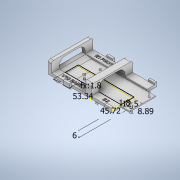
# Autodesk Inventor part: R1 Proto V10 Base
Saved by Autodesk Inventor 2021 (Build 250183000, 183)
## iProperties
Created: 2020-06-07
Part Number: R1 Proto V10 Base
Material: Generic
Document SubType Name: Modeling
Designer: andre
Density: 1 g/cm^3
Appearance: Default
Author: andre
## iProperties of the stored document _3DPrint.ipt
Created: 2020-06-07
Part Number: _3DPrint
Material: Generic
Document SubType Name: Modeling
Designer: andre
Density: 1 g/cm^3
Appearance: Default
Author: andre
Autodesk Inventor part; units mm, degrees
ref_plane "YZ Plane" through (0, 0, 0) normal (1, 0, 0) x (0, 1, 0)
ref_plane "XZ Plane" through (0, 0, 0) normal (0, 1, 0) x (-1, 0, 0)
ref_plane "XY Plane" through (0, 0, 0) normal (0, 0, 1) x (1, 0, 0)
sketch "Sketch1" plane through (0, 0, 0) normal (0, 1, 0) x (-1, 0, 0)
  line L0 (0, 0) -> (62, 0)
  line L1 (62, 0) -> (62, -19.7)
  line L2 (62, -19.7) -> (0, -19.7)
  line L3 (0, -19.7) -> (0, 0)
  dimension "d5" = 62
  dimension "d6" = 19.7
  constraints: 8 end point, 2 parallel, 1 horizontal, 1 perpendicular
  measures "d5" distance of L1.end L2.end
  measures "d6" distance of L0.end L1.end
extrude "Extrusion1" add sketch "Sketch1" along normal blind 2.4
sketch "Sketch3" plane through (-62, 0, 0) normal (0, 0, 1) x (1, 0, 0)
  line L0 (62, 2.4) -> (0, 2.4) projected
  line L1 (62, 0) -> (0, 0) projected
  line L2 (62, 2.4) -> (56, 2.4)
  line L3 (56, 2.4) -> (56, 0)
  line L4 (56, 0) -> (62, 0)
  line L5 (62, 0) -> (62, 2.4)
  line L6 (22, 2.4) -> (22, 0) construction
  line L7 (22, 2.4) -> (16, 2.4)
  line L8 (16, 2.4) -> (16, 0)
  line L9 (16, 0) -> (22, 0)
  line L10 (22, 0) -> (22, 2.4)
  point P0 (62, 0)
  point P1 (22, 0)
  dimension "d9" = 6
  dimension "d13" = 6
  dimension "d14" = 34
  dimension "d79" = 2.4
  constraints: 18 end point, 4 parallel, 4 point on line, 3 perpendicular, 2 horizontal
  measures "d9" distance of L4.end L3.end
  measures "d13" distance of L9.end L8.end
  measures "d14" distance between parallel lines of L3 L6
  measures "d79" distance between parallel lines of L1 L0
extrude "Extrusion2" add sketch "Sketch3" along normal blind 2 contours L5 L1 L3 L0 | L10 L1 L8 L0
ref_plane "Work Plane1" through (0, 0, -19.7) normal (0, 0, -1) x (-1, 0, 0)
sketch "Sketch4" plane through (0, 2.4, 0) normal (0, 1, 0) x (1, 0, 0)
  line L0 (-6, -2) -> (0, -2) projected
  line L1 (-6, -2) -> (0, -2)
  line L2 (0, -2) -> (0, 0)
  line L3 (0, 0) -> (-6, 0)
  line L4 (-6, 0) -> (-6, -2)
  line L5 (-46, -2) -> (-40, -2) projected
  line L6 (-40, 0) -> (-40, -2) projected
  line L7 (-46, -2) -> (-40, -2)
  line L8 (-40, -2) -> (-40, 0)
  line L9 (-40, 0) -> (-46, 0)
  line L10 (-46, 0) -> (-46, -2)
  constraints: 16 end point, 4 parallel, 2 horizontal, 2 perpendicular
extrude "Extrusion3" add sketch "Sketch4" along normal blind 1.6
sketch "Sketch5" plane through (0, 2.4, 0) normal (0, 1, 0) x (1, 0, 0)
  point P0 (0, 0)
sketch "Sketch6" plane through (0, 2.4, 0) normal (0, 1, 0) x (1, 0, 0)
  line L0 (0, 19.7) -> (-62, 19.7) projected
  line L1 (-40, 0) -> (-6, 0) projected
  line L2 (-21, 19.7) -> (-27, 19.7)
  line L3 (-27, 19.7) -> (-27, 0)
  line L4 (-27, 0) -> (-21, 0)
  line L5 (-21, 0) -> (-21, 19.7)
  line L6 (0, 19.7) -> (0, 0) projected
  dimension "d18" = 6
  dimension "d19" = 21
  constraints: 8 end point, 2 parallel, 2 point on line, 1 horizontal, 1 perpendicular
  measures "d18" distance of L4.end L3.end
  measures "d19" distance between parallel lines of L6 L5
extrude "Extrusion4" add sketch "Sketch6" along normal blind 9.6
sketch "Sketch7" plane through (-21, 2.4, 0) normal (1, 0, 0) x (0, 0, -1)
  point P0 (0, -2.4)
sketch "Sketch8" plane through (-21, 2.4, 0) normal (1, 0, 0) x (0, 0, -1)
  line L0 (19.7, 0) -> (19.7, 9.6) projected
  line L1 (19.7, 0) -> (7.2, 0)
  line L2 (7.2, 0) -> (7.2, 8.1)
  line L3 (7.2, 8.1) -> (19.7, 8.1)
  line L4 (19.7, 8.1) -> (19.7, 0)
  line L5 (0, 0) -> (0, 9.6) projected
  line L6 (19.7, 0) -> (0, 0) projected
  line L7 (0, 9.6) -> (19.7, 9.6) projected
  point P0 (0, -2.4)
  point P1 (19.7, 8.1)
  dimension "d22" = 19.7
  dimension "d23" = 9.6
  dimension "d24" = 12.5
  dimension "d25" = 8.1
  constraints: 8 end point, 2 parallel, 1 horizontal, 1 perpendicular
  measures "d22" distance between parallel lines of L0 L5
  measures "d23" distance between parallel lines of L6 L7
  measures "d24" distance between parallel lines of L0 L2
  measures "d25" distance between parallel lines of L1 L3
extrude "Extrusion5" cut sketch "Sketch8" against normal blind 37.6 contours L1 L2 L3 L0
ref_plane "Work Plane2" through (-43, 0, -19.7) normal (-1, 0, 0) x (0, 0, 1)
mirror "Mirror2" about plane through (-43, 0, -19.7) normal (-1, 0, 0) of "Extrusion4", "Extrusion5"
sketch "Sketch12" plane through (0, 2.4, 0) normal (0, 1, 0) x (1, 0, 0)
  line L0 (0, 19.7) -> (0, -2) projected
  line L1 (0, 19.7) -> (-53.34, 19.7)
  line L2 (-53.34, 19.7) -> (-53.34, 7.2)
  line L3 (-53.34, 7.2) -> (0, 7.2)
  line L4 (0, 7.2) -> (0, 19.7)
  point P0 (0, 0)
  point P1 (0, 7.2)
  dimension "d41" = 53.34
  dimension "d42" = 12.5
  constraints: 8 end point, 2 parallel, 1 horizontal, 1 perpendicular
  measures "d41" distance between parallel lines of L2 L0
  measures "d42" distance between parallel lines of L1 L3
extrude "Extrusion8" cut sketch "Sketch12" against normal blind 1.4
fillet "Fillet3" radius 2 2 edges at (-62, 12, 0) (-24, 12, 0) curvature continuous yes
fillet "Fillet4" radius 7 2 edges at (-62, 10.5, -7.2) (-24, 10.5, -7.2) curvature continuous yes
sketch "Sketch13" plane through (0, 1, 0) normal (0, 1, 0) x (1, 0, 0)
  circle A0 centre (6, 10.81) radius 0.9
  circle A1 centre (-39.72, 12.1417) radius 0.9
  line L0 (-53.34, 19.7) -> (0, 19.7) projected
  line L1 (0, 19.7) -> (0, 7.2) projected
  point P0 (0, 0)
  dimension "d48" = 1.8
  dimension "d49" = 1.8
  dimension "d50" = 45.72
  dimension "d51" = 8.89
  dimension "d76" = 6
  constraints: 2 centre point
  measures "d48" diameter of A0
  measures "d49" diameter of A1
  measures "d50" horizontal distance of A1.centre A0.centre
  measures "d51" distance from line of L0 A0.centre
  measures "d76" distance from line of L1 A0.centre
extrude "Extrusion9" add sketch "Sketch13" along normal blind 4 contours A0
mirror "Mirror3" about plane through (0, 0, -19.7) normal (0, 0, -1) of "Extrusion4", "Extrusion5", "Mirror2", "Fillet4", "Fillet3", "Extrusion1", "Extrusion3", "Extrusion2", "Extrusion9", "Extrusion8"
sketch "Sketch14" plane through (-62, 0, 0) normal (-1, 0, 0) x (0, 0, 1)
  line L0 (-58.5888, -16.4354) -> (8.8289, -16.4354)
  line L1 (8.8289, -16.4354) -> (8.8289, 25.7982)
  line L2 (8.8289, 25.7982) -> (-58.5888, 25.7982)
  line L3 (-58.5888, 25.7982) -> (-58.5888, -16.4354)
  point P0 (0, 0)
  constraints: 8 end point, 2 parallel, 1 horizontal, 1 perpendicular
extrude "Extrusion10" cut sketch "Sketch14" along normal blind 5
chamfer "Chamfer1" distance 5 distance2 1.4 1 edges at (-53.34, 2.4, -19.7) measured on face at (-53.84, 2.4, -19.7)
sketch "Sketch15" plane through (0, 2.4, 0) normal (0, 1, 0) x (1, 0, 0)
  line L0 (-57, 38.4) -> (-29, 38.4) construction
  line L1 (-29, 38.4) -> (-29, 33.2) construction
  line L2 (-29, 33.2) -> (-57, 33.2) construction
  line L3 (-57, 33.2) -> (-57, 38.4) construction
  line L4 (-59, 37.4) -> (-59, 2) projected
  line L5 (-27, 2) -> (-27, 37.4) projected
  line L6 (-59, 39.4) -> (-46, 39.4) projected
  line L7 (-58.34, 32.2) -> (0, 32.2) projected
  line L8 (-57, 6.2) -> (-29, 6.2) construction
  line L9 (-29, 6.2) -> (-29, 1) construction
  line L10 (-29, 1) -> (-57, 1) construction
  line L11 (-57, 1) -> (-57, 6.2) construction
  line L12 (0, 7.2) -> (-58.34, 7.2) projected
  line L13 (-59, 0) -> (-46, 0) projected
  line L14 (-14.9129, 6.2) -> (-6.0871, 6.2) construction
  line L15 (-6.0871, 6.2) -> (-6.0871, 1) construction
  line L16 (-6.0871, 1) -> (-14.9129, 1) construction
  line L17 (-14.9129, 1) -> (-14.9129, 6.2) construction
  line L18 (-21, 2) -> (-21, 37.4) projected
  line L19 (0, 7.2) -> (0, 0) projected
  spline S0 degree 2 poles (-51.0157, 2.1) (-50.8394, 2.1) (-50.6147, 2.2691) (-50.5495, 2.4527) knots 0 0 0 1 2 2 2
  line L20 (-50.5495, 2.4527) -> (-49.7307, 4.6556)
  spline S1 degree 2 poles (-49.7307, 4.6556) (-49.7017, 4.7377) (-49.7017, 4.8174) knots 0 0 0 1 1 1
  spline S2 degree 2 poles (-49.7017, 4.8174) (-49.7041, 4.9454) (-49.8732, 5.0976) (-50.0157, 5.1) knots 0 0 0 1 2 2 2
  spline S3 degree 2 poles (-50.0157, 5.1) (-50.1341, 5.1) (-50.279, 4.9865) (-50.3176, 4.8657) knots 0 0 0 1 2 2 2
  line L21 (-50.3176, 4.8657) -> (-50.9988, 2.7691)
  line L22 (-50.9988, 2.7691) -> (-51.0133, 2.7691)
  line L23 (-51.0133, 2.7691) -> (-51.6969, 4.8585)
  spline S4 degree 2 poles (-51.6969, 4.8585) (-51.7331, 4.9841) (-51.8853, 5.1) (-52.0085, 5.1) knots 0 0 0 1 2 2 2
  spline S5 degree 2 poles (-52.0085, 5.1) (-52.1558, 5.0976) (-52.3273, 4.9406) (-52.3297, 4.8101) knots 0 0 0 1 2 2 2
  spline S6 degree 2 poles (-52.3297, 4.8101) (-52.3297, 4.7232) (-52.3007, 4.6386) knots 0 0 0 1 1 1
  line L24 (-52.3007, 4.6386) -> (-51.4867, 2.4551)
  spline S7 degree 2 poles (-51.4867, 2.4551) (-51.4215, 2.2691) (-51.1944, 2.1) (-51.0157, 2.1) knots 0 0 0 1 2 2 2
  spline S8 degree 2 poles (-48.3708, 2.0952) (-48.2331, 2.0976) (-48.0713, 2.2618) (-48.0688, 2.4019) knots 0 0 0 1 2 2 2
  line L25 (-48.0688, 2.4019) -> (-48.0688, 4.7618)
  spline S9 degree 2 poles (-48.0688, 4.7618) (-48.0713, 4.9213) (-48.2524, 5.1024) (-48.4167, 5.1048) knots 0 0 0 1 2 2 2
  spline S10 degree 2 poles (-48.4167, 5.1048) (-48.5085, 5.1048) (-48.6751, 5.0589) (-48.779, 4.9889) knots 0 0 0 1 2 2 2
  line L26 (-48.779, 4.9889) -> (-49.3587, 4.5879)
  spline S11 degree 2 poles (-49.3587, 4.5879) (-49.4287, 4.5372) (-49.4915, 4.4285) (-49.4915, 4.3585) knots 0 0 0 1 2 2 2
  spline S12 degree 2 poles (-49.4915, 4.3585) (-49.4891, 4.2594) (-49.3708, 4.1411) (-49.2766, 4.1411) knots 0 0 0 1 2 2 2
  spline S13 degree 2 poles (-49.2766, 4.1411) (-49.2307, 4.1411) (-49.1558, 4.1652) (-49.1147, 4.1942) knots 0 0 0 1 2 2 2
  line L27 (-49.1147, 4.1942) -> (-48.6872, 4.4937)
  line L28 (-48.6872, 4.4937) -> (-48.6751, 4.4937)
  line L29 (-48.6751, 4.4937) -> (-48.6751, 2.4019)
  spline S14 degree 2 poles (-48.6751, 2.4019) (-48.6727, 2.2618) (-48.5085, 2.0976) (-48.3708, 2.0952) knots 0 0 0 1 2 2 2
  spline S15 degree 2 poles (-46.2597, 2.0734) (-45.8877, 2.0758) (-45.3563, 2.4478) (-45.0713, 3.1314) (-45.0688, 3.6072) knots 0 0 0 1 2 3 3 3
  spline S16 degree 2 poles (-45.0688, 3.6072) (-45.0713, 4.0807) (-45.3563, 4.7594) (-45.8901, 5.1242) (-46.2597, 5.1266) knots 0 0 0 1 2 3 3 3
  spline S17 degree 2 poles (-46.2597, 5.1266) (-46.6292, 5.1242) (-47.163, 4.757) (-47.4505, 4.0783) (-47.4505, 3.6048) knots 0 0 0 1 2 3 3 3
  spline S18 degree 2 poles (-47.4505, 3.6048) (-47.4505, 3.129) (-47.163, 2.4454) (-46.6316, 2.0758) (-46.2597, 2.0734) knots 0 0 0 1 2 3 3 3
  spline S19 degree 2 poles (-46.2597, 2.5638) (-46.5326, 2.5662) (-46.8273, 3.1) (-46.8297, 3.6048) knots 0 0 0 1 2 2 2
  spline S20 degree 2 poles (-46.8297, 3.6048) (-46.8273, 4.1048) (-46.5278, 4.6338) (-46.2597, 4.6362) knots 0 0 0 1 2 2 2
  spline S21 degree 2 poles (-46.2597, 4.6362) (-45.9891, 4.6338) (-45.692, 4.1048) (-45.6896, 3.6048) knots 0 0 0 1 2 2 2
  spline S22 degree 2 poles (-45.6896, 3.6048) (-45.692, 3.1) (-45.9867, 2.5662) (-46.2597, 2.5638) knots 0 0 0 1 2 2 2
  line L30 (-43.535, 2.1386) -> (-42.5471, 2.1386)
  spline S23 degree 2 poles (-42.5471, 2.1386) (-42.0737, 2.1435) (-41.5423, 2.5855) (-41.5374, 2.9744) knots 0 0 0 1 2 2 2
  spline S24 degree 2 poles (-41.5374, 2.9744) (-41.5423, 3.2691) (-41.9215, 3.6531) (-42.2258, 3.6821) knots 0 0 0 1 2 2 2
  line L31 (-42.2258, 3.6821) -> (-42.2258, 3.6966)
  spline S25 degree 2 poles (-42.2258, 3.6966) (-41.9867, 3.7377) (-41.6824, 4.0855) (-41.6775, 4.3319) knots 0 0 0 1 2 2 2
  spline S26 degree 2 poles (-41.6775, 4.3319) (-41.68, 4.67) (-42.1534, 5.0565) (-42.5688, 5.0589) knots 0 0 0 1 2 2 2
  line L32 (-42.5688, 5.0589) -> (-43.535, 5.0589)
  spline S27 degree 2 poles (-43.535, 5.0589) (-43.68, 5.0589) (-43.8394, 4.8923) (-43.8394, 4.7425) knots 0 0 0 1 2 2 2
  line L33 (-43.8394, 4.7425) -> (-43.8394, 2.4575)
  spline S28 degree 2 poles (-43.8394, 2.4575) (-43.8394, 2.3053) (-43.68, 2.1386) (-43.535, 2.1386) knots 0 0 0 1 2 2 2
  line L34 (-43.2283, 2.5952) -> (-43.2283, 3.443)
  line L35 (-43.2283, 3.443) -> (-42.7162, 3.443)
  spline S29 degree 2 poles (-42.7162, 3.443) (-42.4457, 3.4406) (-42.1606, 3.228) (-42.1606, 3.0227) knots 0 0 0 1 2 2 2
  spline S30 degree 2 poles (-42.1606, 3.0227) (-42.1606, 2.8126) (-42.4384, 2.5952) (-42.7041, 2.5952) knots 0 0 0 1 2 2 2
  line L36 (-42.7041, 2.5952) -> (-43.2283, 2.5952)
  line L37 (-43.2283, 3.844) -> (-43.2283, 4.6048)
  line L38 (-43.2283, 4.6048) -> (-42.7283, 4.6048)
  spline S31 degree 2 poles (-42.7283, 4.6048) (-42.5109, 4.6024) (-42.279, 4.4116) (-42.279, 4.2353) knots 0 0 0 1 2 2 2
  spline S32 degree 2 poles (-42.279, 4.2353) (-42.279, 4.0493) (-42.5447, 3.8464) (-42.7911, 3.844) knots 0 0 0 1 2 2 2
  line L39 (-42.7911, 3.844) -> (-43.2283, 3.844)
  spline S33 degree 2 poles (-40.994, 2.1) (-40.8732, 2.1) (-40.7258, 2.2304) (-40.6848, 2.3754) knots 0 0 0 1 2 2 2
  line L40 (-40.6848, 2.3754) -> (-40.5302, 2.8319)
  line L41 (-40.5302, 2.8319) -> (-39.4771, 2.8319)
  line L42 (-39.4771, 2.8319) -> (-39.3225, 2.3705)
  spline S34 degree 2 poles (-39.3225, 2.3705) (-39.2814, 2.228) (-39.1316, 2.1) (-39.0036, 2.1) knots 0 0 0 1 2 2 2
  spline S35 degree 2 poles (-39.0036, 2.1) (-38.8684, 2.1024) (-38.7017, 2.2594) (-38.6993, 2.3874) knots 0 0 0 1 2 2 2
  spline S36 degree 2 poles (-38.6993, 2.3874) (-38.6993, 2.4333) (-38.7162, 2.5227) (-38.7379, 2.5831) knots 0 0 0 1 2 2 2
  line L43 (-38.7379, 2.5831) -> (-39.5399, 4.7546)
  spline S37 degree 2 poles (-39.5399, 4.7546) (-39.6027, 4.9333) (-39.8273, 5.1) (-40.006, 5.1) knots 0 0 0 1 2 2 2
  spline S38 degree 2 poles (-40.006, 5.1) (-40.1775, 5.1) (-40.4022, 4.9309) (-40.465, 4.7546) knots 0 0 0 1 2 2 2
  line L44 (-40.465, 4.7546) -> (-41.2621, 2.5831)
  spline S39 degree 2 poles (-41.2621, 2.5831) (-41.2838, 2.5251) (-41.3031, 2.4261) (-41.3031, 2.3874) knots 0 0 0 1 2 2 2
  spline S40 degree 2 poles (-41.3031, 2.3874) (-41.3031, 2.2546) (-41.1389, 2.1024) (-40.994, 2.1) knots 0 0 0 1 2 2 2
  line L45 (-40.3973, 3.3053) -> (-40.0181, 4.501)
  line L46 (-40.0181, 4.501) -> (-40.0036, 4.501)
  line L47 (-40.0036, 4.501) -> (-39.6171, 3.3053)
  line L48 (-39.6171, 3.3053) -> (-40.3973, 3.3053)
  spline S41 degree 2 poles (-37.2597, 2.0903) (-36.7089, 2.0952) (-36.0882, 2.5879) (-36.0833, 3.0203) knots 0 0 0 1 2 2 2
  spline S42 degree 2 poles (-36.0833, 3.0203) (-36.0809, 3.3512) (-36.5085, 3.7473) (-36.9698, 3.8367) knots 0 0 0 1 2 2 2
  line L49 (-36.9698, 3.8367) -> (-37.279, 3.8995)
  spline S43 degree 2 poles (-37.279, 3.8995) (-37.535, 3.9502) (-37.7669, 4.1266) (-37.7645, 4.2594) knots 0 0 0 1 2 2 2
  spline S44 degree 2 poles (-37.7645, 4.2594) (-37.7597, 4.4237) (-37.4915, 4.6145) (-37.2621, 4.6169) knots 0 0 0 1 2 2 2
  spline S45 degree 2 poles (-37.2621, 4.6169) (-37.0737, 4.6169) (-36.7983, 4.4696) (-36.7258, 4.3053) knots 0 0 0 1 2 2 2
  spline S46 degree 2 poles (-36.7258, 4.3053) (-36.6751, 4.2111) (-36.535, 4.1242) (-36.4336, 4.1242) knots 0 0 0 1 2 2 2
  spline S47 degree 2 poles (-36.4336, 4.1242) (-36.3152, 4.1266) (-36.1751, 4.2594) (-36.1727, 4.3681) knots 0 0 0 1 2 2 2
  spline S48 degree 2 poles (-36.1727, 4.3681) (-36.1727, 4.4092) (-36.1848, 4.4744) (-36.1944, 4.5058) knots 0 0 0 1 2 2 2
  spline S49 degree 2 poles (-36.1944, 4.5058) (-36.2959, 4.7932) (-36.8563, 5.1072) (-37.2621, 5.1097) knots 0 0 0 1 2 2 2
  spline S50 degree 2 poles (-37.2621, 5.1097) (-37.5882, 5.1072) (-38.0906, 4.8874) (-38.3732, 4.4913) (-38.378, 4.2208) knots 0 0 0 1 2 3 3 3
  spline S51 degree 2 poles (-38.378, 4.2208) (-38.378, 3.8947) (-37.9457, 3.4792) (-37.5085, 3.3923) knots 0 0 0 1 2 2 2
  line L50 (-37.5085, 3.3923) -> (-37.1993, 3.3319)
  spline S52 degree 2 poles (-37.1993, 3.3319) (-36.9263, 3.2763) (-36.692, 3.0976) (-36.6944, 2.9551) knots 0 0 0 1 2 2 2
  spline S53 degree 2 poles (-36.6944, 2.9551) (-36.6993, 2.7908) (-36.9964, 2.5855) (-37.2452, 2.5831) knots 0 0 0 1 2 2 2
  spline S54 degree 2 poles (-37.2452, 2.5831) (-37.4577, 2.5807) (-37.7742, 2.7401) (-37.849, 2.9068) knots 0 0 0 1 2 2 2
  spline S55 degree 2 poles (-37.849, 2.9068) (-37.9022, 3.001) (-38.0374, 3.0855) (-38.1292, 3.0831) knots 0 0 0 1 2 2 2
  spline S56 degree 2 poles (-38.1292, 3.0831) (-38.25, 3.0831) (-38.3973, 2.9382) (-38.3998, 2.815) knots 0 0 0 1 2 2 2
  spline S57 degree 2 poles (-38.3998, 2.815) (-38.3998, 2.7739) (-38.3829, 2.6894) (-38.3659, 2.6507) knots 0 0 0 1 2 2 2
  spline S58 degree 2 poles (-38.3659, 2.6507) (-38.2766, 2.4068) (-37.7138, 2.0952) (-37.2597, 2.0903) knots 0 0 0 1 2 2 2
  line L51 (-35.407, 2.1386) -> (-34.0181, 2.1386)
  spline S59 degree 2 poles (-34.0181, 2.1386) (-33.8901, 2.1386) (-33.7428, 2.2715) (-33.7403, 2.3923) knots 0 0 0 1 2 2 2
  spline S60 degree 2 poles (-33.7403, 2.3923) (-33.7428, 2.5106) (-33.8925, 2.6435) (-34.0181, 2.6435) knots 0 0 0 1 2 2 2
  line L52 (-34.0181, 2.6435) -> (-35.1002, 2.6435)
  line L53 (-35.1002, 2.6435) -> (-35.1002, 3.3826)
  line L54 (-35.1002, 3.3826) -> (-34.0713, 3.3826)
  spline S61 degree 2 poles (-34.0713, 3.3826) (-33.9529, 3.3826) (-33.8176, 3.5058) (-33.8152, 3.6169) knots 0 0 0 1 2 2 2
  spline S62 degree 2 poles (-33.8152, 3.6169) (-33.8176, 3.7256) (-33.9553, 3.8512) (-34.0713, 3.8512) knots 0 0 0 1 2 2 2
  line L55 (-34.0713, 3.8512) -> (-35.1002, 3.8512)
  line L56 (-35.1002, 3.8512) -> (-35.1002, 4.5541)
  line L57 (-35.1002, 4.5541) -> (-34.0181, 4.5541)
  spline S63 degree 2 poles (-34.0181, 4.5541) (-33.8925, 4.5541) (-33.7428, 4.687) (-33.7403, 4.8053) knots 0 0 0 1 2 2 2
  spline S64 degree 2 poles (-33.7403, 4.8053) (-33.7428, 4.9261) (-33.8901, 5.0589) (-34.0181, 5.0589) knots 0 0 0 1 2 2 2
  line L58 (-34.0181, 5.0589) -> (-35.407, 5.0589)
  spline S65 degree 2 poles (-35.407, 5.0589) (-35.5519, 5.0589) (-35.7114, 4.8923) (-35.7114, 4.7425) knots 0 0 0 1 2 2 2
  line L59 (-35.7114, 4.7425) -> (-35.7114, 2.4575)
  spline S66 degree 2 poles (-35.7114, 2.4575) (-35.7114, 2.3053) (-35.5519, 2.1386) (-35.407, 2.1386) knots 0 0 0 1 2 2 2
  spline S67 degree 2 poles (-52.1534, 34.2952) (-52.0085, 34.2976) (-51.849, 34.4618) (-51.8466, 34.614) knots 0 0 0 1 2 2 2
  line L60 (-51.8466, 34.614) -> (-51.8466, 35.4063)
  line L61 (-51.8466, 35.4063) -> (-51.3273, 35.4063)
  line L62 (-51.3273, 35.4063) -> (-50.8418, 34.5271)
  spline S68 degree 2 poles (-50.8418, 34.5271) (-50.7717, 34.3966) (-50.6365, 34.2928) (-50.5302, 34.2952) knots 0 0 0 1 2 2 2
  spline S69 degree 2 poles (-50.5302, 34.2952) (-50.3949, 34.2976) (-50.2258, 34.4522) (-50.221, 34.5754) knots 0 0 0 1 2 2 2
  spline S70 degree 2 poles (-50.221, 34.5754) (-50.221, 34.6261) (-50.25, 34.7227) (-50.2862, 34.7855) knots 0 0 0 1 2 2 2
  line L63 (-50.2862, 34.7855) -> (-50.7089, 35.515)
  spline S71 degree 2 poles (-50.7089, 35.515) (-50.465, 35.6213) (-50.2065, 36.0512) (-50.2065, 36.329) knots 0 0 0 1 2 2 2
  spline S72 degree 2 poles (-50.2065, 36.329) (-50.2089, 36.7662) (-50.7548, 37.2541) (-51.2621, 37.2589) knots 0 0 0 1 2 2 2
  line L64 (-51.2621, 37.2589) -> (-52.1534, 37.2589)
  spline S73 degree 2 poles (-52.1534, 37.2589) (-52.2983, 37.2589) (-52.4577, 37.0923) (-52.4577, 36.9425) knots 0 0 0 1 2 2 2
  line L65 (-52.4577, 36.9425) -> (-52.4577, 34.614)
  spline S74 degree 2 poles (-52.4577, 34.614) (-52.4577, 34.4618) (-52.2983, 34.2976) (-52.1534, 34.2952) knots 0 0 0 1 2 2 2
  line L66 (-51.8466, 35.8507) -> (-51.8466, 36.7807)
  line L67 (-51.8466, 36.7807) -> (-51.3273, 36.7807)
  spline S75 degree 2 poles (-51.3273, 36.7807) (-51.0978, 36.7783) (-50.837, 36.5319) (-50.8345, 36.3169) knots 0 0 0 1 2 2 2
  spline S76 degree 2 poles (-50.8345, 36.3169) (-50.8345, 36.0971) (-51.0882, 35.8531) (-51.3225, 35.8507) knots 0 0 0 1 2 2 2
  line L68 (-51.3225, 35.8507) -> (-51.8466, 35.8507)
  spline S77 degree 2 poles (-48.8104, 34.2952) (-48.6727, 34.2976) (-48.5109, 34.4618) (-48.5085, 34.6019) knots 0 0 0 1 2 2 2
  line L69 (-48.5085, 34.6019) -> (-48.5085, 36.9618)
  spline S78 degree 2 poles (-48.5085, 36.9618) (-48.5109, 37.1213) (-48.692, 37.3024) (-48.8563, 37.3048) knots 0 0 0 1 2 2 2
  spline S79 degree 2 poles (-48.8563, 37.3048) (-48.9481, 37.3048) (-49.1147, 37.2589) (-49.2186, 37.1889) knots 0 0 0 1 2 2 2
  line L70 (-49.2186, 37.1889) -> (-49.7983, 36.7879)
  spline S80 degree 2 poles (-49.7983, 36.7879) (-49.8684, 36.7372) (-49.9312, 36.6285) (-49.9312, 36.5585) knots 0 0 0 1 2 2 2
  spline S81 degree 2 poles (-49.9312, 36.5585) (-49.9287, 36.4594) (-49.8104, 36.3411) (-49.7162, 36.3411) knots 0 0 0 1 2 2 2
  spline S82 degree 2 poles (-49.7162, 36.3411) (-49.6703, 36.3411) (-49.5954, 36.3652) (-49.5543, 36.3942) knots 0 0 0 1 2 2 2
  line L71 (-49.5543, 36.3942) -> (-49.1268, 36.6937)
  line L72 (-49.1268, 36.6937) -> (-49.1147, 36.6937)
  line L73 (-49.1147, 36.6937) -> (-49.1147, 34.6019)
  spline S83 degree 2 poles (-49.1147, 34.6019) (-49.1123, 34.4618) (-48.9481, 34.2976) (-48.8104, 34.2952) knots 0 0 0 1 2 2 2
  spline S84 degree 2 poles (-46.692, 34.3) (-46.5471, 34.3024) (-46.3877, 34.4667) (-46.3853, 34.6188) knots 0 0 0 1 2 2 2
  line L74 (-46.3853, 34.6188) -> (-46.3853, 35.2589)
  line L75 (-46.3853, 35.2589) -> (-45.8394, 35.2589)
  spline S85 degree 2 poles (-45.8394, 35.2589) (-45.5302, 35.2614) (-45.0616, 35.5101) (-44.7983, 35.957) (-44.7983, 36.2589) knots 0 0 0 1 2 3 3 3
  spline S86 degree 2 poles (-44.7983, 36.2589) (-44.7983, 36.5609) (-45.0543, 37.0101) (-45.5085, 37.2565) (-45.8104, 37.2589) knots 0 0 0 1 2 3 3 3
  line L76 (-45.8104, 37.2589) -> (-46.692, 37.2589)
  spline S87 degree 2 poles (-46.692, 37.2589) (-46.837, 37.2589) (-46.9964, 37.0923) (-46.9964, 36.9425) knots 0 0 0 1 2 2 2
  line L77 (-46.9964, 36.9425) -> (-46.9964, 34.6188)
  spline S88 degree 2 poles (-46.9964, 34.6188) (-46.9964, 34.4667) (-46.837, 34.3024) (-46.692, 34.3) knots 0 0 0 1 2 2 2
  line L78 (-46.3853, 35.7372) -> (-46.3853, 36.7758)
  line L79 (-46.3853, 36.7758) -> (-45.9722, 36.7758)
  spline S89 degree 2 poles (-45.9722, 36.7758) (-45.7065, 36.7734) (-45.4215, 36.5077) (-45.4191, 36.2565) knots 0 0 0 1 2 2 2
  spline S90 degree 2 poles (-45.4191, 36.2565) (-45.4215, 36.0053) (-45.7089, 35.7396) (-45.9722, 35.7372) knots 0 0 0 1 2 2 2
  line L80 (-45.9722, 35.7372) -> (-46.3853, 35.7372)
  spline S91 degree 2 poles (-44.1316, 34.2952) (-43.9867, 34.2976) (-43.8273, 34.4618) (-43.8249, 34.614) knots 0 0 0 1 2 2 2
  line L81 (-43.8249, 34.614) -> (-43.8249, 35.4063)
  line L82 (-43.8249, 35.4063) -> (-43.3056, 35.4063)
  line L83 (-43.3056, 35.4063) -> (-42.82, 34.5271)
  spline S92 degree 2 poles (-42.82, 34.5271) (-42.75, 34.3966) (-42.6147, 34.2928) (-42.5085, 34.2952) knots 0 0 0 1 2 2 2
  spline S93 degree 2 poles (-42.5085, 34.2952) (-42.3732, 34.2976) (-42.2041, 34.4522) (-42.1993, 34.5754) knots 0 0 0 1 2 2 2
  spline S94 degree 2 poles (-42.1993, 34.5754) (-42.1993, 34.6261) (-42.2283, 34.7227) (-42.2645, 34.7855) knots 0 0 0 1 2 2 2
  line L84 (-42.2645, 34.7855) -> (-42.6872, 35.515)
  spline S95 degree 2 poles (-42.6872, 35.515) (-42.4432, 35.6213) (-42.1848, 36.0512) (-42.1848, 36.329) knots 0 0 0 1 2 2 2
  spline S96 degree 2 poles (-42.1848, 36.329) (-42.1872, 36.7662) (-42.7331, 37.2541) (-43.2403, 37.2589) knots 0 0 0 1 2 2 2
  line L85 (-43.2403, 37.2589) -> (-44.1316, 37.2589)
  spline S97 degree 2 poles (-44.1316, 37.2589) (-44.2766, 37.2589) (-44.436, 37.0923) (-44.436, 36.9425) knots 0 0 0 1 2 2 2
  line L86 (-44.436, 36.9425) -> (-44.436, 34.614)
  spline S98 degree 2 poles (-44.436, 34.614) (-44.436, 34.4618) (-44.2766, 34.2976) (-44.1316, 34.2952) knots 0 0 0 1 2 2 2
  line L87 (-43.8249, 35.8507) -> (-43.8249, 36.7807)
  line L88 (-43.8249, 36.7807) -> (-43.3056, 36.7807)
  spline S99 degree 2 poles (-43.3056, 36.7807) (-43.0761, 36.7783) (-42.8152, 36.5319) (-42.8128, 36.3169) knots 0 0 0 1 2 2 2
  spline S100 degree 2 poles (-42.8128, 36.3169) (-42.8128, 36.0971) (-43.0664, 35.8531) (-43.3007, 35.8507) knots 0 0 0 1 2 2 2
  line L89 (-43.3007, 35.8507) -> (-43.8249, 35.8507)
  spline S101 degree 2 poles (-40.4674, 34.2903) (-40.0326, 34.2928) (-39.4022, 34.6575) (-39.0616, 35.3314) (-39.0592, 35.7976) knots 0 0 0 1 2 3 3 3
  spline S102 degree 2 poles (-39.0592, 35.7976) (-39.0616, 36.2662) (-39.4022, 36.9425) (-40.0326, 37.3072) (-40.4674, 37.3097) knots 0 0 0 1 2 3 3 3
  spline S103 degree 2 poles (-40.4674, 37.3097) (-40.9022, 37.3072) (-41.5326, 36.9425) (-41.8732, 36.2662) (-41.8756, 35.7976) knots 0 0 0 1 2 3 3 3
  spline S104 degree 2 poles (-41.8756, 35.7976) (-41.8732, 35.3314) (-41.5326, 34.6575) (-40.9022, 34.2928) (-40.4674, 34.2903) knots 0 0 0 1 2 3 3 3
  spline S105 degree 2 poles (-40.4674, 34.8) (-40.8321, 34.8048) (-41.2476, 35.3338) (-41.2524, 35.7976) knots 0 0 0 1 2 2 2
  spline S106 degree 2 poles (-41.2524, 35.7976) (-41.2476, 36.2638) (-40.8297, 36.7952) (-40.4674, 36.8) knots 0 0 0 1 2 2 2
  spline S107 degree 2 poles (-40.4674, 36.8) (-40.1051, 36.7952) (-39.6872, 36.2638) (-39.6848, 35.7976) knots 0 0 0 1 2 2 2
  spline S108 degree 2 poles (-39.6848, 35.7976) (-39.6872, 35.3338) (-40.1051, 34.8048) (-40.4674, 34.8) knots 0 0 0 1 2 2 2
  spline S109 degree 2 poles (-37.663, 34.3) (-37.5181, 34.3024) (-37.3587, 34.4667) (-37.3563, 34.6188) knots 0 0 0 1 2 2 2
  line L90 (-37.3563, 34.6188) -> (-37.3563, 36.7541)
  line L91 (-37.3563, 36.7541) -> (-36.7524, 36.7541)
  spline S110 degree 2 poles (-36.7524, 36.7541) (-36.6268, 36.7541) (-36.4795, 36.887) (-36.4771, 37.0053) knots 0 0 0 1 2 2 2
  spline S111 degree 2 poles (-36.4771, 37.0053) (-36.4771, 37.1261) (-36.6268, 37.2589) (-36.7524, 37.2589) knots 0 0 0 1 2 2 2
  line L92 (-36.7524, 37.2589) -> (-38.5713, 37.2589)
  spline S112 degree 2 poles (-38.5713, 37.2589) (-38.6993, 37.2589) (-38.8466, 37.1261) (-38.849, 37.0053) knots 0 0 0 1 2 2 2
  spline S113 degree 2 poles (-38.849, 37.0053) (-38.8466, 36.887) (-38.6969, 36.7541) (-38.5713, 36.7541) knots 0 0 0 1 2 2 2
  line L93 (-38.5713, 36.7541) -> (-37.9674, 36.7541)
  line L94 (-37.9674, 36.7541) -> (-37.9674, 34.6188)
  spline S114 degree 2 poles (-37.9674, 34.6188) (-37.9674, 34.4667) (-37.808, 34.3024) (-37.663, 34.3) knots 0 0 0 1 2 2 2
  spline S115 degree 2 poles (-34.8563, 34.2903) (-34.4215, 34.2928) (-33.7911, 34.6575) (-33.4505, 35.3314) (-33.4481, 35.7976) knots 0 0 0 1 2 3 3 3
  spline S116 degree 2 poles (-33.4481, 35.7976) (-33.4505, 36.2662) (-33.7911, 36.9425) (-34.4215, 37.3072) (-34.8563, 37.3097) knots 0 0 0 1 2 3 3 3
  spline S117 degree 2 poles (-34.8563, 37.3097) (-35.2911, 37.3072) (-35.9215, 36.9425) (-36.2621, 36.2662) (-36.2645, 35.7976) knots 0 0 0 1 2 3 3 3
  spline S118 degree 2 poles (-36.2645, 35.7976) (-36.2621, 35.3314) (-35.9215, 34.6575) (-35.2911, 34.2928) (-34.8563, 34.2903) knots 0 0 0 1 2 3 3 3
  spline S119 degree 2 poles (-34.8563, 34.8) (-35.221, 34.8048) (-35.6365, 35.3338) (-35.6413, 35.7976) knots 0 0 0 1 2 2 2
  spline S120 degree 2 poles (-35.6413, 35.7976) (-35.6365, 36.2638) (-35.2186, 36.7952) (-34.8563, 36.8) knots 0 0 0 1 2 2 2
  spline S121 degree 2 poles (-34.8563, 36.8) (-34.494, 36.7952) (-34.0761, 36.2638) (-34.0737, 35.7976) knots 0 0 0 1 2 2 2
  spline S122 degree 2 poles (-34.0737, 35.7976) (-34.0761, 35.3338) (-34.494, 34.8048) (-34.8563, 34.8) knots 0 0 0 1 2 2 2
  line L95 (-12.5278, 2.106) -> (-11.5399, 2.106)
  spline S123 degree 2 poles (-11.5399, 2.106) (-11.0664, 2.1109) (-10.535, 2.5529) (-10.5302, 2.9418) knots 0 0 0 1 2 2 2
  spline S124 degree 2 poles (-10.5302, 2.9418) (-10.535, 3.2365) (-10.9143, 3.6205) (-11.2186, 3.6495) knots 0 0 0 1 2 2 2
  line L96 (-11.2186, 3.6495) -> (-11.2186, 3.664)
  spline S125 degree 2 poles (-11.2186, 3.664) (-10.9795, 3.7051) (-10.6751, 4.0529) (-10.6703, 4.2993) knots 0 0 0 1 2 2 2
  spline S126 degree 2 poles (-10.6703, 4.2993) (-10.6727, 4.6374) (-11.1461, 5.0239) (-11.5616, 5.0263) knots 0 0 0 1 2 2 2
  line L97 (-11.5616, 5.0263) -> (-12.5278, 5.0263)
  spline S127 degree 2 poles (-12.5278, 5.0263) (-12.6727, 5.0263) (-12.8321, 4.8597) (-12.8321, 4.7099) knots 0 0 0 1 2 2 2
  line L98 (-12.8321, 4.7099) -> (-12.8321, 2.4249)
  spline S128 degree 2 poles (-12.8321, 2.4249) (-12.8321, 2.2727) (-12.6727, 2.106) (-12.5278, 2.106) knots 0 0 0 1 2 2 2
  line L99 (-12.221, 2.5626) -> (-12.221, 3.4104)
  line L100 (-12.221, 3.4104) -> (-11.7089, 3.4104)
  spline S129 degree 2 poles (-11.7089, 3.4104) (-11.4384, 3.408) (-11.1534, 3.1954) (-11.1534, 2.9901) knots 0 0 0 1 2 2 2
  spline S130 degree 2 poles (-11.1534, 2.9901) (-11.1534, 2.78) (-11.4312, 2.5626) (-11.6969, 2.5626) knots 0 0 0 1 2 2 2
  line L101 (-11.6969, 2.5626) -> (-12.221, 2.5626)
  line L102 (-12.221, 3.8114) -> (-12.221, 4.5722)
  line L103 (-12.221, 4.5722) -> (-11.721, 4.5722)
  spline S131 degree 2 poles (-11.721, 4.5722) (-11.5036, 4.5698) (-11.2717, 4.379) (-11.2717, 4.2027) knots 0 0 0 1 2 2 2
  spline S132 degree 2 poles (-11.2717, 4.2027) (-11.2717, 4.0167) (-11.5374, 3.8138) (-11.7838, 3.8114) knots 0 0 0 1 2 2 2
  line L104 (-11.7838, 3.8114) -> (-12.221, 3.8114)
  line L105 (-9.9336, 2.106) -> (-8.3176, 2.106)
  spline S133 degree 2 poles (-8.3176, 2.106) (-8.1969, 2.1085) (-8.064, 2.2389) (-8.064, 2.35) knots 0 0 0 1 2 2 2
  spline S134 degree 2 poles (-8.064, 2.35) (-8.064, 2.4611) (-8.1969, 2.5915) (-8.3176, 2.5915) knots 0 0 0 1 2 2 2
  line L106 (-8.3176, 2.5915) -> (-9.4191, 2.5915)
  line L107 (-9.4191, 2.5915) -> (-9.4191, 2.6036)
  line L108 (-9.4191, 2.6036) -> (-8.7862, 3.2123)
  spline S135 degree 2 poles (-8.7862, 3.2123) (-8.5495, 3.4345) (-8.2621, 3.7655) (-8.1341, 4.0674) (-8.1341, 4.2413) knots 0 0 0 1 2 3 3 3
  spline S136 degree 2 poles (-8.1341, 4.2413) (-8.1365, 4.4949) (-8.3949, 4.8766) (-8.8587, 5.0891) (-9.1703, 5.0915) knots 0 0 0 1 2 3 3 3
  spline S137 degree 2 poles (-9.1703, 5.0915) (-9.4481, 5.0891) (-9.8684, 4.9128) (-10.1389, 4.6302) (-10.1896, 4.4659) knots 0 0 0 1 2 3 3 3
  spline S138 degree 2 poles (-10.1896, 4.4659) (-10.1993, 4.4345) (-10.2114, 4.3693) (-10.2114, 4.3355) knots 0 0 0 1 2 2 2
  spline S139 degree 2 poles (-10.2114, 4.3355) (-10.2114, 4.2196) (-10.0737, 4.0867) (-9.9505, 4.0867) knots 0 0 0 1 2 2 2
  spline S140 degree 2 poles (-9.9505, 4.0867) (-9.8539, 4.0843) (-9.7283, 4.1737) (-9.68, 4.263) knots 0 0 0 1 2 2 2
  spline S141 degree 2 poles (-9.68, 4.263) (-9.6002, 4.4394) (-9.3539, 4.6157) (-9.1775, 4.6157) knots 0 0 0 1 2 2 2
  spline S142 degree 2 poles (-9.1775, 4.6157) (-8.9771, 4.6133) (-8.7331, 4.3862) (-8.7307, 4.2027) knots 0 0 0 1 2 2 2
  spline S143 degree 2 poles (-8.7307, 4.2027) (-8.7283, 4.1012) (-8.8056, 3.9104) (-9.0036, 3.6761) (-9.1824, 3.5046) knots 0 0 0 1 2 3 3 3
  line L109 (-9.1824, 3.5046) -> (-10.0543, 2.6737)
  spline S144 degree 2 poles (-10.0543, 2.6737) (-10.1461, 2.5891) (-10.2234, 2.4514) (-10.221, 2.3669) knots 0 0 0 1 2 2 2
  spline S145 degree 2 poles (-10.221, 2.3669) (-10.221, 2.251) (-10.0785, 2.1085) (-9.9336, 2.106) knots 0 0 0 1 2 2 2
  dimension "d59" = 2
  dimension "d60" = 2
  dimension "d61" = 1
  dimension "d62" = 1
  dimension "d63" = 1
  dimension "d64" = 1
  dimension "d65" = 2
  dimension "d66" = 2
  dimension "d69" = 0
  dimension "d70" = 0
  dimension "d71" = 6.0871
  dimension "d72" = 6.0871
  constraints: 6 other
  measures "d59" distance between parallel lines of L4 L3
  measures "d60" distance between parallel lines of L5 L1
  measures "d61" distance between parallel lines of L6 L0
  measures "d62" distance between parallel lines of L7 L2
  measures "d63" distance between parallel lines of L12 L8
  measures "d64" distance between parallel lines of L13 L10
  measures "d65" distance between parallel lines of L4 L11
  measures "d66" distance between parallel lines of L5 L9
  measures "d69" distance between parallel lines of L14 L8
  measures "d70" distance between parallel lines of L16 L10
  measures "d71" distance between parallel lines of L18 L17
  measures "d72" distance between parallel lines of L19 L15
extrude "Extrusion11" cut sketch "Sketch15" against normal blind 1 contours S7 L24 S6 S5 S4 L23 L22 L21 S3 S2 S1 L20 S0 | S14 L29 L28 L27 S13 S12 S11 L26 S10 S9 L25 S8 | S18 S17 S16 S15 | S28 L33 S27 L32 S26 S25 L31 S24 S23 L30 | S40 S39 L44 S38 S37 L43 S36 S35 S34 L42 L41 L40 S33 | S58 S57 S56 S55 S54 S53 S52 L50 S51 S50 S49 S48 S47 S46 S45 S44 S43 L49 S42 S41 | S66 L59 S65 L58 S64 S63 L57 L56 L55 S62 S61 L54 L53 L52 S60 S59 L51 | S74 L65 S73 L64 S72 S71 L63 S70 S69 S68 L62 L61 L60 S67 | S83 L73 L72 L71 S82 S81 S80 L70 S79 S78 L69 S77 | S88 L77 S87 L76 S86 S85 L75 L74 S84 | S98 L86 S97 L85 S96 S95 L84 S94 S93 S92 L83 L82 L81 S91 | S104 S103 S102 S101 | S114 L94 L93 S113 S112 L92 S111 S110 L91 L90 S109 | S118 S117 S116 S115 | S128 L98 S127 L97 S126 S125 L96 S124 S123 L95 | S145 S144 L109 S143 S142 S141 S140 S139 S138 S137 S136 S135 L108 L107 L106 S134 S133 L105
sketch "Sketch16" plane through (0, 0, 2) normal (1, 0, 0) x (0, 0, -1)
  line L0 (34.2, 1) -> (9.2, 1) projected
  line L1 (2, 0) -> (41.4, 0) projected
  line L2 (9.2, 1) -> (34.2, 1)
  line L3 (34.2, 1) -> (34.2, 0)
  line L4 (34.2, 0) -> (9.2, 0)
  line L5 (9.2, 0) -> (9.2, 1)
  point P0 (9.2, 0)
  dimension "d73" = 25
  constraints: 8 end point, 2 parallel, 1 horizontal, 1 perpendicular, 1 point on line
  measures "d73" distance of L3.end L4.end
extrude "Extrusion12" add sketch "Sketch16" along normal blind 8
extrude "Extrusion13" add sketch "Sketch13" along normal blind 1 contours A1
mirror "Mirror4" about plane through (0, 0, -19.7) normal (0, 0, -1) of "Extrusion13"
equation "\"d24\" = d22 + d42 - d6"
equation "\"d49\" = d48"
equation "\"d60\" = d59"
equation "\"d62\" = d61"
equation "\"d63\" = d61"
equation "\"d64\" = d61"
equation "\"d65\" = d59"
equation "\"d66\" = d59"
equation "\"d72\" = d71"
equation "\"d73\" = 2 * d42"
equation "\"d29\" = -d30"
equation "\"d30\" = 19"
body "Solid1"
